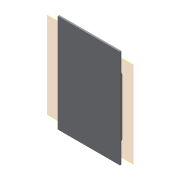
# Autodesk Inventor part: 01_Zeiss_Axiotech_adapterplate
Saved by Autodesk Inventor 2019 (Build 230136000, 136)
## iProperties
Created: 2019-05-02
Part Number: 01_Zeiss_Axiotech_adapterplate
Material: Generic
Document SubType Name: Modeling
Designer: diederichbenedict
Density: 1 g/cm^3
Appearance: Default
Author: diederichbenedict
Autodesk Inventor part; units mm, degrees
ref_plane "YZ Plane" through (0, 0, 0) normal (1, 0, 0) x (0, 1, 0)
ref_plane "XZ Plane" through (0, 0, 0) normal (0, 1, 0) x (-1, 0, 0)
ref_plane "XY Plane" through (0, 0, 0) normal (0, 0, 1) x (1, 0, 0)
ref_plane "Work Plane1" through (0, 0, 0) normal (0, 0, 1) x (1, 0, 0)
sketch "Sketch1" plane through (0, 0, 0) normal (0, 0, 1) x (1, 0, 0)
  arc A0 (80, 65) -> (65, 80) centre (65, 65) ccw projected
  line L0 (80, 65) -> (80, -65) projected
  arc A1 (65, -80) -> (80, -65) centre (65, -65) ccw projected
  line L1 (65, -80) -> (-65, -80) projected
  arc A2 (-80, -65) -> (-65, -80) centre (-65, -65) ccw projected
  line L2 (-80, -65) -> (-80, 65) projected
  arc A3 (-65, 80) -> (-80, 65) centre (-65, 65) ccw projected
  line L3 (-65, 80) -> (65, 80) projected
  line L4 (-100, -100) -> (100, -100) projected
  line L5 (100, -100) -> (100, 100) projected
  line L6 (100, 100) -> (-100, 100) projected
  line L7 (-100, 100) -> (-100, -100) projected
  line L8 (79, -65) -> (79, 65)
  arc A4 (79, 65) -> (65, 79) centre (65, 65) ccw
  line L9 (65, 79) -> (-65, 79)
  arc A5 (-65, 79) -> (-79, 65) centre (-65, 65) ccw
  line L10 (-79, 65) -> (-79, -65)
  arc A6 (-79, -65) -> (-65, -79) centre (-65, -65) ccw
  line L11 (-65, -79) -> (65, -79)
  arc A7 (65, -79) -> (79, -65) centre (65, -65) ccw
  point P0 (0, 0)
  dimension "d0" = 1
  constraints: 8 end point, 8 point on circle, 4 centre point, 7 other
  measures "d0" distance between parallel lines of L0 L8
extrude "Extrusion1" add sketch "Sketch1" against normal blind 2 contours A7 L11 A6 L10 A5 L9 A4 L8
sketch "Sketch2" plane through (0, 0, 0) normal (0, 0, 1) x (1, 0, 0)
  line L0 (79, -65) -> (79, 65) projected
  arc A0 (79, 65) -> (65, 79) centre (65, 65) ccw projected
  line L1 (65, 79) -> (-65, 79) projected
  arc A1 (-65, 79) -> (-79, 65) centre (-65, 65) ccw projected
  line L2 (-79, 65) -> (-79, -65) projected
  arc A2 (-79, -65) -> (-65, -79) centre (-65, -65) ccw projected
  line L3 (-65, -79) -> (65, -79) projected
  arc A3 (65, -79) -> (79, -65) centre (65, -65) ccw projected
  line L4 (-79, -125) -> (79, -125)
  line L5 (79, -125) -> (79, 125)
  line L6 (79, 125) -> (-79, 125)
  line L7 (-79, 125) -> (-79, -125)
  line L8 (-79, -125) -> (79, 125) construction
  line L9 (79, -125) -> (-79, 125) construction
  point P0 (0, 0)
  dimension "d3" = 250
  constraints: 12 end point, 2 midpoint, 2 parallel, 1 horizontal, 1 perpendicular
  measures "d3" distance of L5.end L4.end
extrude "Extrusion2" add sketch "Sketch2" along normal blind 4
body "Solid1"
